rod_label_clip (Autodesk Fusion 360 design; units mm, degrees)
part number: 2026-09-05-07-00-16-324
Autodesk Fusion 360 part; units mm, degrees
sketch "Ring" plane through (0, 0, 0) normal (0, 1, 0) x (1, 0, 0)
  circle A0 centre (0, 0) radius 17.05
  circle A1 centre (0, 0) radius 19.45
  dimension "d234" = 34.1
  dimension "d235" = 38.9
  constraint coincident A0.centre A1.centre
  constraint concentric A0 A1
  measures "d234" diameter of A0
  measures "d235" diameter of A1
extrude "Ring (1)" add sketch "Ring" along normal mid plane 20
sketch "Mouth" plane through (0, 0, 0) normal (0, 1, 0) x (1, 0, 0)
  line L0 (0, 0) -> (42.3486, -24.45)
  line L1 (42.3486, -24.45) -> (0, -48.9)
  line L2 (0, -48.9) -> (-42.3486, -24.45)
  line L3 (-42.3486, -24.45) -> (0, 0)
  line L4 (0, 0) -> (0, -48.9) construction
  dimension "d238" = 48.9
  dimension "d239" = 48.9
  dimension "d240" = 48.9
  dimension "d241" = 60
  dimension "d242" = 60
  constraint coincident L0.start L3.end
  constraint vertical L4
  constraint coincident L1.end L2.start
  measures "d238" distance of L0.start L0.end
  measures "d239" distance of L0.start L2.end
  measures "d240" distance of L0.start L1.end
  measures "d241" angle of L0 L4
  measures "d242" angle of L3 L4
extrude "Mouth (1)" cut sketch "Mouth" along normal mid plane 30
ref_plane "WorkPlane3" through (0, 12.125, 0) normal (-0.173648, 0, -0.984808) x (0, 1, 0)
sketch "Stem section" plane through (0, 0, 0) normal (-0.173648, 0, -0.984808) x (0, 1, 0)
  line L0 (1.75, 0) -> (22.5, 0) construction
  line L1 (-10, 1.2) -> (10, 1.2)
  line L2 (10, 1.2) -> (10, -1.2)
  line L3 (10, -1.2) -> (-10, -1.2)
  line L4 (-10, -1.2) -> (-10, 1.2)
  line L5 (0, 0) -> (0, 4.8) construction
  dimension "d247" = 2.4
  dimension "d248" = 4.8
  dimension "d249" = 20
  constraint parallel L0 L1
  constraint parallel L0 L3
  constraint perpendicular L0 L4
  constraint perpendicular L0 L2
  constraint symmetric L0 L1 L3
  constraint coincident L5.start origin
  constraint perpendicular L0 L5
  constraint symmetric L2 L4 L5
  measures "d247" distance of L1 L3
  measures "d248" distance of L5.start L5.end
  measures "d249" distance of L2 L4
extrude "Stem" add sketch "Stem section" along normal blind 12.7 from surface at 18.25
sketch "Face section" plane through (0, 0, 0) normal (-0.173648, 0, -0.984808) x (0, 1, 0)
  line L0 (1.75, 0) -> (22.5, 0) construction
  line L1 (-10, 1.2) -> (48, 1.2)
  line L2 (48, 1.2) -> (48, -1.2)
  line L3 (48, -1.2) -> (-10, -1.2)
  line L4 (-10, -1.2) -> (-10, 1.2)
  line L5 (-10, -1.2) -> (-10, 1.2) construction
  dimension "d253" = 2.4
  dimension "d254" = 58
  constraint parallel L0 L1
  constraint parallel L0 L3
  constraint perpendicular L0 L4
  constraint perpendicular L0 L2
  constraint symmetric L0 L1 L3
  constraint collinear L4 L5
  measures "d253" distance of L1 L3
  measures "d254" distance of L2 L4
extrude "Label face" add sketch "Face section" along normal blind 29 from surface at 30.95
equation "clipWidth = 20.0 mm" comment "ring and stem width along the rod"
equation "faceWidth = 58.0 mm" comment "label face width along the rod"
equation "rodOuterDiameter = 33.4 mm" comment "rod the clip snaps onto"
equation "clipClearance = 0.7 mm" comment "diametral, so the clip slides"
equation "clipWall = 2.4 mm" comment "ring wall thickness"
equation "mouthHalfAngleDeg = 60.0 deg" comment "half the mouth opening"
equation "paddleThickness = 2.4 mm" comment "stem and label face thickness"
equation "stemEndRadius = ( rodOuterDiameter + clipClearance + 2 * clipWall ) / 2 + stemLength" comment "derived: stem ends, label face begins"
equation "faceEndRadius = stemEndRadius + faceHeight" comment "derived: outer edge of the label face"
equation "paddleAngleDeg = 100.0 deg" comment "paddle drop below horizontal"
equation "stemStartRadius = ( rodOuterDiameter + clipClearance ) / 2 + clipWall / 2" comment "derived: stem starts mid ring wall"
equation "stemLength = 11.5 mm" comment "stem reach beyond the ring outer wall"
equation "faceHeight = 29.0 mm" comment "label face, from stem end outward"
equation "d234 = rodOuterDiameter + clipClearance"
equation "d235 = rodOuterDiameter + clipClearance + 2 * clipWall"
equation "d236 = clipWidth"
equation "d238 = ( ( rodOuterDiameter + clipClearance + 2 * clipWall ) / 2 + 5 mm ) / cos(mouthHalfAngleDeg)"
equation "d239 = ( ( rodOuterDiameter + clipClearance + 2 * clipWall ) / 2 + 5 mm ) / cos(mouthHalfAngleDeg)"
equation "d240 = ( ( rodOuterDiameter + clipClearance + 2 * clipWall ) / 2 + 5 mm ) / cos(mouthHalfAngleDeg)"
equation "d241 = mouthHalfAngleDeg"
equation "d242 = mouthHalfAngleDeg"
equation "d243 = clipWidth + 10 mm"
equation "d245 = paddleAngleDeg"
equation "d247 = paddleThickness"
equation "d248 = paddleThickness * 2"
equation "d249 = clipWidth"
equation "d250 = stemStartRadius"
equation "d251 = stemEndRadius - stemStartRadius"
equation "d253 = paddleThickness"
equation "d254 = faceWidth"
equation "d255 = stemEndRadius"
equation "d256 = faceEndRadius - stemEndRadius"
named bodies: "rod_label_clip"
